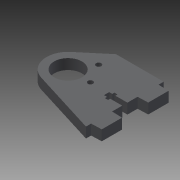
# Autodesk Inventor part: X_wspierak
Saved by Autodesk Inventor 2013 (Build 170138000, 138)
## iProperties
Created: 2013-12-11
Part Number: X_wspierak
Material: Generic
Document SubType Name: Modeling
Designer: dzban
Density: 1 g/cm^3
Author: dzban
Autodesk Inventor part; units mm, degrees
ref_plane "YZ Plane" through (0, 0, 0) normal (1, 0, 0) x (0, 1, 0)
ref_plane "XZ Plane" through (0, 0, 0) normal (0, 1, 0) x (-1, 0, 0)
ref_plane "XY Plane" through (0, 0, 0) normal (0, 0, 1) x (1, 0, 0)
sketch "Sketch1" plane through (0, 0, 0) normal (0, 0, 1) x (1, 0, 0)
  circle A0 centre (0, 0) radius 8.05
  circle A1 centre (13, 0) radius 1.5
  circle A2 centre (6.5, 11.2583) radius 1.5
  line L0 (-12.0771, 21.6) -> (34, 21.6) construction
  line L1 (34, 21.6) -> (34, -16.4745) construction
  line L2 (6.2782, 21.6) -> (34, 21.6)
  line L3 (34, 21.6) -> (34, 18.6)
  line L4 (34, 18.6) -> (40, 18.4)
  line L5 (40, 18.4) -> (40, 6.6)
  line L6 (40, 6.6) -> (34, 6.4)
  line L7 (34, 6.4) -> (34, 0.5)
  line L8 (34, 0.5) -> (27, 0.5)
  line L9 (27, 0.5) -> (27, 1.75)
  line L10 (27, 1.75) -> (25.2, 1.75)
  line L11 (25.2, 1.75) -> (25.2, 0.5)
  line L12 (25.2, 0.5) -> (23.4, 0.5)
  line L13 (23.4, 0.5) -> (23.4, -2.5)
  line L14 (23.4, -2.5) -> (25.2, -2.5)
  line L15 (25.2, -2.5) -> (25.2, -3.75)
  line L16 (25.2, -3.75) -> (27, -3.75)
  line L17 (27, -3.75) -> (27, -2.5)
  line L18 (27, -2.5) -> (34, -2.5)
  line L19 (34, -2.5) -> (34, -8.4)
  line L20 (34, -8.4) -> (40, -8.6)
  line L21 (40, -8.6) -> (40, -20.4)
  line L22 (40, -20.4) -> (34, -20.6)
  line L23 (34, -20.6) -> (34, -23.6)
  arc A3 (-8.0405, 9.5708) -> (-3.6935, -11.9419) centre (0, 0) ccw
  line L24 (34, -23.6) -> (-3.6935, -11.9419)
  line L25 (6.2782, 21.6) -> (-8.0405, 9.5708)
  dimension "d0" = 3
  dimension "d2" = 3
  dimension "d3" = 16.1
  dimension "d4" = 13
  dimension "d5" = 13
  dimension "d6" = 34
  dimension "d7" = 21.6
  dimension "d9" = 3
  dimension "d10" = 1.25
  dimension "d11" = 1.25
  dimension "d12" = 1.8
  dimension "d13" = 1.8
  dimension "d14" = 7
  dimension "d15" = 12.2
  dimension "d16" = 11.8
  dimension "d17" = 0.2
  dimension "d18" = 6
  dimension "d19" = 12.2
  dimension "d20" = 11.8
  dimension "d21" = 0.2
  dimension "d22" = 14.8
  dimension "d23" = 5.9
  dimension "d24" = 3
  dimension "d27" = 60
  dimension "d28" = 3
  dimension "d29" = 25
  constraints: 52 end point, 9 collinear, 4 centre point, 3 horizontal, 3 perpendicular, 3 vertical, 2 coincident, 2 point on circle, 2 point on line, 2 tangent, 1 horizontal alignment, 1 parallel
  measures "d0" diameter of A2
  measures "d2" diameter of A1
  measures "d3" diameter of A0
  measures "d4" distance of point (0, 0) A1.centre
  measures "d5" distance of point (0, 0) A2.centre
  measures "d6" distance from line of L1 point (0, 0)
  measures "d7" distance from line of L0 point (0, 0)
  measures "d9" distance between parallel lines of L8 L18
  measures "d10" distance between parallel lines of L18 L16
  measures "d11" distance between parallel lines of L10 L12
  measures "d12" distance between parallel lines of L11 L13
  measures "d13" distance between parallel lines of L9 L11
  measures "d14" distance between parallel lines of L1 L9
  measures "d15" distance of L3.end L6.end
  measures "d16" distance of L5.end L4.end
  measures "d17" vertical distance of L3.end L4.end
  measures "d18" distance between parallel lines of L3 L5
  measures "d19" distance of L19.end L22.end
  measures "d20" distance of L20.end L21.end
  measures "d21" vertical distance of L21.end L22.end
  measures "d22" distance of L6.end L19.end
  measures "d23" distance of L6.end L7.end
  measures "d24" distance from line of L2 L3.end
  measures "d28" distance of L22.end L23.end
  measures "d29" diameter of A3
extrude "Extrusion1" add sketch "Sketch1" along normal blind 6
body "Solid1"
